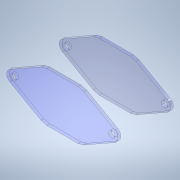
# Autodesk Inventor part: Papa John Mounting Plate with hinge half 2
Saved by Autodesk Inventor 2020 (Build 240168000, 168)
## iProperties
Created: 2020-01-31
Part Number: Papa John Mounting Plate with hinge half 2
Material: Polycarbonate, Clear
Document SubType Name: Modeling
Designer: aidan
Density: 1.2 g/cm^3
Appearance: Polycarbonate - Clear
Author: aidan
Autodesk Inventor part; units mm, degrees
ref_plane "YZ Plane" through (0, 0, 0) normal (1, 0, 0) x (0, 1, 0)
ref_plane "XZ Plane" through (0, 0, 0) normal (0, 1, 0) x (-1, 0, 0)
sketch "Sketch1" plane through (0, 0, 0) normal (0, 0, 1) x (1, 0, 0)
  line L0 (-85.5838, 10.5171) -> (-66.5338, 10.5171)
  line L1 (-66.5338, -39.724) -> (-85.5838, -39.724)
  line L2 (-85.5838, 10.5171) -> (-129.7381, -14.6035)
  line L3 (-129.7381, -14.6035) -> (-85.5838, -39.724)
  line L4 (-85.5838, 10.5171) -> (-85.5838, -39.724) construction
  line L5 (-66.5338, 10.5171) -> (-66.5338, -39.724)
  dimension "d40" = 50.8
  dimension "d41" = 19.05
  constraints: 12 end point, 2 vertical, 1 equal length, 1 horizontal, 1 parallel
  measures "d40" distance of L0.start L2.end
  measures "d41" distance of L0.start L0.end
extrude "Extrusion1" add sketch "Sketch1" along normal blind 2.9972
fillet "Fillet1" radius 6.35 1 edges at (-129.7381, -14.6035, 1.4986)
chamfer "Chamfer1" distance 3.175 angle 45 2 edges at (-85.5838, 10.5171, 1.4986) (-85.5838, -39.724, 1.4986)
sketch "Sketch3" plane through (0, 0, 2.9972) normal (0, 0, 1) x (1, 0, 0)
  arc A0 (-120.0369, -9.0842) -> (-120.0369, -20.1228) centre (-116.8968, -14.6035) ccw projected
  circle A1 centre (-116.8968, -14.6035) radius 3.175
  point P0 (0, 0)
  dimension "d19" = 6.35
  constraints: 1 centre point, 1 coincident
  measures "d19" diameter of A1
hole "Hole1" at (-116.8968, -14.6035, 2.9972) direction (0, 0, -1) diameter 6.35 end through all
ref_plane "Work Plane1" through (0, 0, 28.2194) normal (0, 0, 1) x (1, 0, 0)
mirror "Mirror1" about plane through (0, 0, 28.2194) normal (0, 0, 1) of "Extrusion1", "Fillet1", "Chamfer1", "Hole1"
mirror "Mirror2" about plane through (-66.5338, -39.724, 56.4388) normal (1, 0, 0)
body "Solid1"
